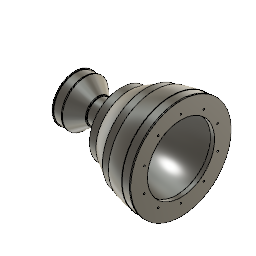
rear_mounting_shaft_eng_model (Autodesk Fusion 360 design; units mm, degrees)
Autodesk Fusion 360 part; units mm, degrees
sketch "Sketch1" plane through (0, 0, 0) normal (0, 1, 0) x (1, 0, 0)
  line L0 (0, 0) -> (253, 0) construction
  line L1 (253, 0) -> (253, -120) construction
  line L2 (0, -120) -> (0, 0) construction
  line L3 (0, -55) -> (2.5, -55)
  line L4 (2.5, -55) -> (2.5, -53)
  line L5 (2.5, -53) -> (22.5, -53)
  line L6 (22.5, -53) -> (22.5, -55)
  line L7 (22.5, -55) -> (25, -55)
  line L8 (22.5, -55) -> (57.5, -55) construction
  line L9 (57.5, -55) -> (57.5, -30) construction
  line L10 (57.5, -30) -> (55, -30)
  line L11 (25, -55) -> (55, -30)
  line L12 (57.5, -30) -> (57.5, -29.7796)
  line L13 (57.5, -29.7796) -> (57.5, -28)
  line L14 (57.5, -28) -> (77.5, -28)
  line L15 (77.5, -28) -> (77.5, -30)
  line L16 (77.5, -30) -> (80, -30)
  line L17 (253, -120) -> (250, -120)
  line L18 (0, -55) -> (0, -30)
  arc A0 (87.5, -23.2906) -> (243, -109.7053) centre (255.0428, 95.0809) ccw
  line L19 (23.7795, -43) -> (51.1319, -20.2063)
  line L20 (10, -43) -> (23.7795, -43)
  line L21 (10, -43) -> (10, -30)
  line L22 (10, -30) -> (0, -30)
  line L23 (51.1319, -20.2063) -> (85.3629, -20.2063)
  line L24 (253, -120) -> (253, -110)
  arc A1 (85.3629, -20.2063) -> (243, -109.7053) centre (255.0428, 95.0809) ccw
  line L25 (253, -110) -> (253, -80)
  line L26 (253, -80) -> (243, -80)
  line L27 (243, -80) -> (243, -109.7053)
  line L28 (230, -118.5966) -> (230, -117.5)
  line L29 (230, -117.5) -> (250, -117.5)
  line L30 (250, -117.5) -> (250, -120)
  line L31 (253, -120) -> (250, -120) construction
  line L32 (230, -120) -> (0, -120) construction
  line L33 (190, -167.9989) -> (190, 64.1278) construction
  line L34 (170, -159.3868) -> (170, 52.862) construction
  line L35 (130, -158.4855) -> (130, 61.424) construction
  line L36 (110, -157.8306) -> (110, 88.7531) construction
  line L37 (358.5261, -104.57) -> (17.8717, -104.57) construction
  line L38 (363.4901, -75.89) -> (29.0407, -75.89) construction
  line L39 (170, -102.5373) -> (170, -104.57)
  line L40 (190, -104.57) -> (170, -104.57)
  arc A2 (190, -109.9914) -> (230, -118.5966) centre (255.0428, 95.0809) ccw
  line L41 (190, -109.9914) -> (190, -104.57)
  line L42 (110, -75.89) -> (130, -75.89)
  line L43 (110, -63.8147) -> (110, -75.89)
  line L44 (130, -75.89) -> (130, -79.9891)
  arc A3 (80, -30) -> (110, -63.8147) centre (255.0428, 95.0809) ccw
  arc A4 (130, -79.9891) -> (170, -102.5373) centre (255.0428, 95.0809) ccw
  dimension "d78" = 120
  dimension "d79" = 253
  dimension "d80" = 55
  dimension "d81" = 2.5
  dimension "d82" = 20
  dimension "d83" = 2
  dimension "d84" = 2
  dimension "d85" = 2.5
  dimension "d86" = 35
  dimension "d87" = 25
  dimension "d88" = 2.5
  dimension "d89" = 20
  dimension "d90" = 2
  dimension "d91" = 2
  dimension "d92" = 2.5
  dimension "d93" = 3
  dimension "d94" = 215.14
  dimension "d95" = 25
  dimension "d97" = 7.7937
  dimension "d98" = 80
  dimension "d99" = 10
  dimension "d100" = 20
  dimension "d101" = 2.5
  dimension "d102" = 40
  dimension "d103" = 20
  dimension "d104" = 40
  dimension "d105" = 20
  dimension "d106" = 75.89
  dimension "d107" = 104.57
  constraint horizontal L0
  constraint vertical L1
  constraint horizontal L31
  constraint vertical L2
  constraint coincident L0.start L2.end
  constraint coincident L2 L3.start
  constraint perpendicular L2 L3
  constraint perpendicular L3 L4
  constraint perpendicular L4 L5
  constraint perpendicular L5 L6
  constraint perpendicular L6 L7
  constraint perpendicular L2 L8
  constraint perpendicular L5 L9
  constraint perpendicular L9 L10
  constraint perpendicular L10 L13
  constraint perpendicular L13 L14
  constraint perpendicular L14 L15
  constraint perpendicular L15 L16
  constraint perpendicular L1 L17
  constraint coincident L2 L18.end
  constraint concentric A0 A3
  constraint perpendicular L21 L22
  constraint horizontal L23
  constraint concentric A0 A1
  constraint coincident L1 L25.end
  constraint parallel L1 L25
  constraint perpendicular L25 L26
  constraint perpendicular L27 L31
  constraint vertical L28
  constraint horizontal L29
  constraint vertical L30
  constraint collinear L31 L32
  constraint perpendicular L0 L33
  constraint vertical L34
  constraint vertical L35
  constraint perpendicular L0 L36
  constraint horizontal L37
  constraint horizontal L38
  constraint coincident L34 L39.start
  constraint coincident L34 L39.end
  constraint coincident L37 L39.end
  constraint coincident L37 L40.start
  constraint coincident L33 L40.start
  constraint coincident L33 A2.start
  constraint concentric A2 A3
  constraint coincident L36 L42.start
  constraint coincident L38 L42.start
  constraint coincident L35 L42.end
  constraint coincident L38 L42.end
  constraint coincident L36 L43.start
  constraint coincident L44.end A3
  constraint coincident L35 L44.end
  constraint concentric A3 A4
  measures "d78" distance of L0.end L1.end
  measures "d79" distance of L1.end L2.start
  measures "d80" distance of L0 L3
  measures "d81" distance of L3.start L3.end
  measures "d82" distance of L4.end L5.end
  measures "d83" distance of L5.end L6.end
  measures "d84" distance of L3.end L4.end
  measures "d85" distance of L6.end L7.end
  measures "d86" distance of L6.end L8.end
  measures "d87" distance of L8.end L9.end
  measures "d88" distance of L9.end L10.end
  measures "d89" distance of L13.end L14.end
  measures "d90" distance of L14.end L15.end
  measures "d91" distance of L9.end L13.end
  measures "d92" distance of L15.end L16.end
  measures "d93" distance of L1.end L17.end
  measures "d94" radius of A3
  measures "d95" distance of L3.start L18.end
  measures "d97" distance of L14 L23
  measures "d98" distance of L0.end L25.end
  measures "d99" distance of L25.end L26.end
  measures "d100" distance of L28.end L29.end
  measures "d101" distance of L17.end L29.end
  measures "d102" distance of L28.end L33
  measures "d103" distance of L33 L34
  measures "d104" distance of L34 L35
  measures "d105" distance of L35 L36
  measures "d106" distance of L0 L38
  measures "d107" distance of L0 L37
revolve "Revolve3" add sketch "Sketch1" angle 360 about axis through (0, 0, 0) along (1, 0, 0)
sketch "Sketch6" plane through (253, 0, 0) normal (1, 0, 0) x (0, 1, 0)
  circle A0 centre (0, 0) radius 80
  circle A1 centre (0, 0) radius 120
  line L0 (0, 0) -> (0, 205.4416) construction
  circle A2 centre (0, 92) radius 2
  dimension "d109" = 4
  dimension "d110" = 92
  constraint coincident A0.centre A1.centre
  constraint vertical L0
  constraint coincident L0 A2.centre
  measures "d109" diameter of A2
  measures "d110" distance of A0.centre A2.centre
extrude "Extrude3" cut sketch "Sketch6" along normal mid plane 30 contours A2
pattern_circular "C-Pattern3" count 10 over 360 about axis through (1.75, 0, 0) along (1, 0, 0) of "Extrude3"
sketch "Sketch7" plane through (0, 0, 0) normal (-1, 0, 0) x (0, -1, 0)
  circle A0 centre (0, 0) radius 55
  circle A1 centre (0, 0) radius 30
  line L0 (0, 0) -> (0, 179.9785) construction
  circle A2 centre (0, 47.5) radius 2
  dimension "d115" = 4
  dimension "d116" = 47.5
  constraint coincident A0.centre A1.centre
  constraint vertical L0
  constraint coincident L0 A2.centre
  measures "d115" diameter of A2
  measures "d116" distance of A0.centre A2.centre
extrude "Extrude4" cut sketch "Sketch7" along normal mid plane 20 contours A2
pattern_circular "C-Pattern4" count 10 over 360 about axis through (1.75, 0, 0) along (1, 0, 0) of "Extrude4"
